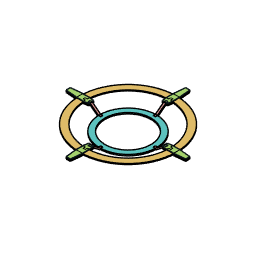
シロコ_ヘイロー_mk2 v9 (Autodesk Fusion 360 design; units mm, degrees)
Autodesk Fusion 360 part; units mm, degrees
sketch "スケッチ1" plane through (0, 0, 0) normal (0, 0, 1) x (1, 0, 0) in component "outer_ring"
  circle A0 centre (0, 0) radius 100
  circle A1 centre (0, 0) radius 116
  line L0 (-105, 2.5) -> (-105, -2.5)
  line L1 (0, 0) -> (-116, 0) construction
  line L2 (-105, 2.5) -> (-99.9687, 2.5)
  line L3 (-105, -2.5) -> (-99.9687, -2.5)
  line L4 (-2.5, -105) -> (-2.5, -99.9687)
  line L5 (-2.5, -105) -> (2.5, -105)
  line L6 (2.5, -105) -> (2.5, -99.9687)
  line L7 (105, -2.5) -> (99.9687, -2.5)
  line L8 (105, -2.5) -> (105, 2.5)
  line L9 (105, 2.5) -> (99.9687, 2.5)
  line L10 (2.5, 105) -> (2.5, 99.9687)
  line L11 (2.5, 105) -> (-2.5, 105)
  line L12 (-2.5, 105) -> (-2.5, 99.9687)
  point P0 (-100, 0)
  dimension "d1" = 200
  dimension "d2" = 232
  dimension "d14" = 5
  dimension "d15" = 5
  dimension "d17" = 360
  constraint coincident A0.centre A1.centre
  constraint concentric A0 A1
  constraint vertical L0
  constraint coincident A1 L1.end
  constraint perpendicular L0 L1
  constraint coincident A0 L2.end
  constraint perpendicular L0 L2
  constraint coincident A0 L3.end
  constraint perpendicular L0 L3
  constraint symmetric L1 L2 L3
  constraint coincident L1 P0
  constraint coincident A0 P0
  measures "d1" diameter of A0
  measures "d2" diameter of A1
  measures "d14" distance of L0.start L0.end
  measures "d15" distance of L0 P0
extrude "押し出し2" add sketch "スケッチ1" along normal blind 2 makes body 1 in component "outer_ring"
ref_plane "作業平面1" through (0, 0, -15) normal (0, 0, 1) x (1, 0, 0) in component "inner_ring"
sketch "スケッチ1 (2)" plane through (0, 0, -15) normal (0, 0, 1) x (1, 0, 0) in component "inner_ring"
  circle A0 centre (0, 0) radius 55
  circle A1 centre (0, 0) radius 68
  line L0 (0, 0) -> (-68, 0) construction
  line L1 (-63, 2.5) -> (-63, -2.5)
  line L2 (-63, 2.5) -> (-67.954, 2.5)
  line L3 (-63, -2.5) -> (-67.954, -2.5)
  line L4 (-2.5, -63) -> (-2.5, -67.954)
  line L5 (-2.5, -63) -> (2.5, -63)
  line L6 (2.5, -63) -> (2.5, -67.954)
  line L7 (63, -2.5) -> (67.954, -2.5)
  line L8 (63, -2.5) -> (63, 2.5)
  line L9 (63, 2.5) -> (67.954, 2.5)
  line L10 (2.5, 63) -> (2.5, 67.954)
  line L11 (2.5, 63) -> (-2.5, 63)
  line L12 (-2.5, 63) -> (-2.5, 67.954)
  dimension "d6" = 110
  dimension "d7" = 136
  dimension "d8" = 5
  dimension "d9" = 5
  dimension "d11" = 360
  constraint coincident A0.centre A1.centre
  constraint concentric A0 A1
  constraint coincident A1 L0.end
  constraint horizontal L0
  constraint perpendicular L0 L1
  constraint coincident A1 L2.end
  constraint perpendicular L1 L2
  constraint coincident A1 L3.end
  constraint perpendicular L1 L3
  constraint symmetric L0 L2 L3
  measures "d6" diameter of A0
  measures "d7" diameter of A1
  measures "d8" distance of L1.start L1.end
  measures "d9" distance of L0.end L1
extrude "押し出し1" add sketch "スケッチ1 (2)" along normal blind 2 separate body contours A1 L1 L2 L3 L4 L5 L6 L7 L8 L9 L10 L11 L12 makes body 2 in component "inner_ring"
sketch "スケッチ1 (3)" plane through (0, 0, 2) normal (0, 0, 1) x (-1, 0, 0) in component "protrusion_front"
  line L0 (2.5, -105) -> (-2.5, -105)
  line L1 (-2.5, -105) -> (-2.5, -99.9687)
  arc A0 (-99.9687, -2.5) -> (-2.5, -99.9687) centre (0, 0) ccw
  line L2 (-99.9687, -2.5) -> (-105, -2.5)
  line L3 (-105, -2.5) -> (-105, 2.5)
  line L4 (-105, 2.5) -> (-99.9687, 2.5)
  arc A1 (-2.5, 99.9687) -> (-99.9687, 2.5) centre (0, 0) ccw
  line L5 (-2.5, 99.9687) -> (-2.5, 105)
  line L6 (-2.5, 105) -> (2.5, 105)
  line L7 (2.5, 105) -> (2.5, 99.9687)
  arc A2 (99.9687, 2.5) -> (2.5, 99.9687) centre (0, 0) ccw
  line L8 (99.9687, 2.5) -> (105, 2.5)
  line L9 (105, 2.5) -> (105, -2.5)
  line L10 (105, -2.5) -> (99.9687, -2.5)
  arc A3 (2.5, -99.9687) -> (99.9687, -2.5) centre (0, 0) ccw
  line L11 (2.5, -99.9687) -> (2.5, -105)
  circle A4 centre (0, 0) radius 116
  line L12 (143, 0) -> (88, 0) construction
  line L13 (0, 0) -> (88, 0) construction
  circle A5 centre (0, 0) radius 116 construction
  circle A6 centre (0, 0) radius 100 construction
  line L14 (143, -5) -> (143, 5)
  line L15 (115.7573, -7.5) -> (115.7573, 7.5) construction
  line L16 (143, -5) -> (115.7573, -7.5)
  line L17 (143, 5) -> (115.7573, 7.5)
  line L18 (88, -6) -> (88, 6)
  line L19 (115.7573, -7.5) -> (99.7184, -7.5)
  line L20 (115.7573, 7.5) -> (99.7184, 7.5)
  line L21 (99.7184, 7.5) -> (88, 6)
  line L22 (99.7184, -7.5) -> (88, -6)
  line L23 (93, -2.5) -> (93, 2.5)
  line L24 (93, -2.5) -> (88, -2.5)
  line L25 (93, 2.5) -> (88, 2.5)
  circle A7 centre (0, 0) radius 99.75
  circle A8 centre (0, 0) radius 116.25
  line L26 (104.9, 2.4462) -> (104.9, -2.4538)
  line L27 (104.9, 2.4462) -> (99.72, 2.4462)
  line L28 (104.9, -2.4538) -> (99.7198, -2.4538)
  dimension "d20" = 55
  dimension "d21" = 88
  dimension "d22" = 232
  dimension "d23" = 200
  dimension "d24" = 10
  dimension "d25" = 15
  dimension "d26" = 12
  dimension "d27" = 5
  dimension "d28" = 5
  dimension "d29" = 199.5
  dimension "d30" = 232.5
  dimension "d33" = 4.9
  dimension "d37" = 104.9
  dimension "d38" = 5.18
  constraint horizontal L12
  constraint coincident A0.centre A1.centre
  constraint horizontal L13
  constraint coincident L12.end L13.end
  constraint concentric A0 A5
  constraint perpendicular L12 L14
  constraint midpoint L12.start L14
  constraint vertical L15
  constraint coincident A5 L15.start
  constraint symmetric L12 L15.start L15.end
  constraint vertical L18
  constraint midpoint L12.end L18
  constraint horizontal L19
  constraint coincident L15.start L16.end
  constraint coincident A6 L19.end
  constraint perpendicular L15 L20
  constraint coincident L15.end L17.end
  constraint coincident A6 L20.end
  constraint vertical L23
  constraint coincident L18 L24.end
  constraint perpendicular L18 L24
  constraint coincident L18 L25.end
  constraint perpendicular L18 L25
  constraint symmetric L12 L24 L25
  constraint concentric A6 A8
  constraint perpendicular L12 L26
  constraint coincident A7 L27.end
  constraint perpendicular L26 L27
  constraint perpendicular L26 L28
  constraint coincident A7 L28.end
  measures "d20" distance of L12.start L12.end
  measures "d21" distance of A0.centre L12.end
  measures "d22" diameter of A5
  measures "d23" diameter of A6
  measures "d24" distance of L14.start L14.end
  measures "d25" distance of L15.start L15.end
  measures "d26" distance of L18.start L18.end
  measures "d27" distance of L23.start L23.end
  measures "d28" distance of L23.start L24.end
  measures "d29" diameter of A7
  measures "d30" diameter of A8
  measures "d33" distance of L26.start L26.end
  measures "d37" distance of A0.centre L26
  measures "d38" distance of L26.start L27.end
extrude "押し出し2'" add sketch "スケッチ1 (3)" along normal blind 1 separate body contours A2 L8 L9 L10 A3 L21 L22 A7 L26 L27 L28 | A2 L8 L9 L10 A3 A4 L19 L20 | A4 L16 L17 A8 | L18 L21 L22 L23 L24 L25 A7 | L14 L16 L17 A8 | A7 L26 L27 L28 picked at (115.8862, 6.6596) makes body 3 in component "protrusion_front"
extrude "押し出し3" add sketch "スケッチ1 (3)" against normal blind 1 contours L18 L21 L22 L23 L24 L25 A7 | L14 L16 L17 A8 bodies 3 in component "protrusion_front"
extrude "押し出し4" add sketch "スケッチ1 (3)" against normal blind 2 contours A7 L26 L27 L28 bodies 3 in component "protrusion_front"
extrude "押し出し1'" add 2 faces at (-134.0744, -0.8313, 1) (-93.49, -5.3227, 1) along direction (0, 0, -1) blind 2 separate body on bodies 3 makes body 4 at (-134.0744, -0.8313, 1) makes body 5 at (-93.49, -5.3227, 1) in component "protrusion_back"
extrude "押し出し2''" cut 2 faces at (-134.0744, -0.8313, 1) (-93.49, -5.3227, 1) along direction (0, 0, -1) blind 1 on bodies 4 5 bodies 4 5 in component "protrusion_back"
loft "ロフト1" add section 1 face at (-99.7465, -0.8306, -0.6667) section 2 face at (-116.1044, -5.8169, -0.3333) on bodies 4 5 bodies 4 5 in component "protrusion_back"
extrude "押し出し3'" add 2 faces at (-134.0744, -0.8313, 1) (-93.49, -5.3227, 1) along direction (0, 0, -1) blind 1 on bodies 3 bodies 4 in component "protrusion_back"
move_body "移動1" bodies 3 to x (1, 0, 0) y (0, 1, 0) z (0, 0, 1) at (0, 0, 0.5) in component "protrusion_front"
extrude "押し出し5" add 2 faces at (-93.49, -5.3227, 1.5) (-134.0744, -0.8313, 1.5) along direction (0, 0, -1) blind 0.5 on bodies 3 bodies 3 in component "protrusion_front"
extrude "押し出し4'" add 2 faces at (-93.49, -5.3227, 1) (-134.0744, -0.8313, 1) along direction (0, 0, 1) blind 0.5 on bodies 4 bodies 4 in component "protrusion_back"
sketch "スケッチ1 (4)" plane through (0, 0, 3.5) normal (0, 0, 1) x (-1, 0, 0) in component "support"
  line L0 (93, -2.5) -> (88, -2.5)
  line L1 (88, -2.5) -> (88, -6)
  line L2 (88, -6) -> (99.7184, -7.5)
  line L3 (99.7184, -7.5) -> (115.7573, -7.5)
  line L4 (115.7573, -7.5) -> (143, -5)
  line L5 (143, -5) -> (143, 5)
  line L6 (143, 5) -> (115.7573, 7.5)
  line L7 (115.7573, 7.5) -> (99.7184, 7.5)
  line L8 (99.7184, 7.5) -> (88, 6)
  line L9 (88, 6) -> (88, 2.5)
  line L10 (88, 2.5) -> (93, 2.5)
  line L11 (93, 2.5) -> (93, -2.5)
  line L12 (93, -2.5) -> (88, -2.5)
  line L13 (88, -2.5) -> (88, 2.5)
  line L14 (88, 2.5) -> (93, 2.5)
  line L15 (93, 2.5) -> (93, -2.5)
  constraint horizontal L12
  constraint vertical L13
  constraint horizontal L14
  constraint vertical L15
  constraint coincident L9.end L10.start
  constraint coincident L0.start L11.end
sketch "スケッチ2" plane through (0, 0, -15) normal (0, 0, -1) x (1, 0, 0) in component "support"
  circle A0 centre (0, 0) radius 55
  line L0 (-2.5, -63) -> (2.5, -63)
  line L1 (2.5, -63) -> (2.5, -67.954)
  arc A1 (2.5, -67.954) -> (67.954, -2.5) centre (0, 0) ccw
  line L2 (67.954, -2.5) -> (63, -2.5)
  line L3 (63, -2.5) -> (63, 2.5)
  line L4 (63, 2.5) -> (67.954, 2.5)
  arc A2 (67.954, 2.5) -> (2.5, 67.954) centre (0, 0) ccw
  line L5 (2.5, 67.954) -> (2.5, 63)
  line L6 (2.5, 63) -> (-2.5, 63)
  line L7 (-2.5, 63) -> (-2.5, 67.954)
  arc A3 (-2.5, 67.954) -> (-67.954, 2.5) centre (0, 0) ccw
  line L8 (-67.954, 2.5) -> (-63, 2.5)
  line L9 (-63, 2.5) -> (-63, -2.5)
  line L10 (-63, -2.5) -> (-67.954, -2.5)
  arc A4 (-67.954, -2.5) -> (-2.5, -67.954) centre (0, 0) ccw
  line L11 (-2.5, -67.954) -> (-2.5, -63)
  line L12 (-67.954, 2.5) -> (-62.954, 2.5)
  line L13 (-62.954, 2.5) -> (-62.954, -2.5)
  line L14 (-62.954, -2.5) -> (-67.954, -2.5)
  line L15 (-67.954, -2.5) -> (-67.954, 2.5)
  dimension "d67" = 5
  dimension "d68" = 5
  constraint horizontal L12
  constraint vertical L13
  constraint horizontal L14
  constraint vertical L15
  constraint coincident A3.end L8.start
  measures "d67" distance of A3.end L12.end
  measures "d68" distance of A3.end L10.end
loft "ロフト1'" add profiles "スケッチ2", "スケッチ1 (4)" section 1 contours L8 L9 L10 L12 L14 L15 section 2 contours L0 L10 L11 L12 L13 L14 L15 separate body makes body 6 in component "support"
sketch "スケッチ1 (5)" plane through (0, 0, 3.5) normal (0, 0, 1) x (-1, 0, 0) in component "protrusion"
  line L0 (93, -2.5) -> (88, -2.5)
  line L1 (88, -2.5) -> (88, -6)
  line L2 (88, -6) -> (99.7184, -7.5)
  line L3 (99.7184, -7.5) -> (115.7573, -7.5)
  line L4 (115.7573, -7.5) -> (143, -5)
  line L5 (143, -5) -> (143, 5)
  line L6 (143, 5) -> (115.7573, 7.5)
  line L7 (115.7573, 7.5) -> (99.7184, 7.5)
  line L8 (99.7184, 7.5) -> (88, 6)
  line L9 (88, 6) -> (88, 2.5)
  line L10 (88, 2.5) -> (93, 2.5)
  line L11 (93, 2.5) -> (93, -2.5)
extrude "押し出し6" add sketch "スケッチ1 (3)" along normal up to surface (1.5 mm away) contours L18 L23 L24 L25 bodies 3 in component "protrusion_front"
extrude "押し出し7" cut 1 faces at (-89.6667, 0.8333, 2) along direction (0, 0, 1) blind 1 on bodies 3 bodies 3 in component "protrusion_front"
extrude "押し出し8" cut 1 faces at (-91.3333, 2.5, 1.6667) along direction (0, 1, 0) blind 0.05 on bodies 3 bodies 3 in component "protrusion_front"
extrude "押し出し9" cut 1 faces at (-89.6667, -2.5, 2.3333) along direction (0, -1, 0) blind 0.05 on bodies 3 bodies 3 in component "protrusion_front"
extrude "押し出し5'" cut 1 faces at (-89.6667, -2.5, -0.1667) along direction (0, -1, 0) blind 0.05 on bodies 4 bodies 4 in component "protrusion_back"
extrude "押し出し6'" cut 1 faces at (-89.6667, 2.5, -0.1667) along direction (0, 1, 0) blind 0.05 on bodies 4 bodies 4 in component "protrusion_back"
sketch "スケッチ1 (6)" plane through (0, 0, 0) normal (0, 1, 0) x (1, 0, 0) in component "pirrer"
  line L0 (-63, 13) -> (-63, 16)
  line L1 (-69.087, 16) -> (-63, 16)
  line L2 (-88, -2.3333) -> (-88, -3)
  line L3 (-88, -3) -> (-93, -3)
  line L4 (-93, -3) -> (-93, 1.5)
  line L5 (-63, 13) -> (-68, 13)
  line L6 (-93, 1.5) -> (-88, 1.5)
  line L7 (-88, 1.5) -> (-69.087, 16)
  line L8 (-88, -2.3333) -> (-68, 13)
  dimension "d88" = 3
  constraint perpendicular L3 L4
  constraint perpendicular L0 L5
  constraint parallel L7 L8
  measures "d88" distance of L0.start L0.end
extrude "押し出し1''" add sketch "スケッチ1 (6)" along normal blind 2.5 separate body makes body 7 in component "pirrer"
extrude "押し出し2'''" add 1 faces at (-81.3333, 0, -4.0556) along direction (0, -1, 0) blind 2.5 on bodies 7 bodies 7 in component "pirrer"
extrude "押し出し2''''" add 1 faces at (9.1157, -61.1473, -15) along direction (0, 0, -1) blind 1 on bodies 2 bodies 2 in component "inner_ring"
component_pattern "component pattern"
component "outer_ring" placed x (1, 0, 0) y (0, 1, 0) z (0, 0, 1) at (0, 0, 0)
component "inner_ring" placed x (1, 0, 0) y (0, 1, 0) z (0, 0, 1) at (0, 0, 0)
component "protrusion" placed x (1, 0, 0) y (0, 1, 0) z (0, 0, 1) at (0, 0, 0)
component "pirrer" placed x (1, 0, 0) y (0, 1, 0) z (0, 0, 1) at (0, 0, 0)
component "protrusion" placed x (0, 1, 0) y (-1, 0, 0) z (0, 0, 1) at (0, 0, 0)
component "pirrer" placed x (0, 1, 0) y (-1, 0, 0) z (0, 0, 1) at (0, 0, 0)
component "protrusion" placed x (-1, 0, 0) y (0, -1, 0) z (0, 0, 1) at (0, 0, 0)
component "pirrer" placed x (-1, 0, 0) y (0, -1, 0) z (0, 0, 1) at (0, 0, 0)
component "protrusion" placed x (0, -1, 0) y (1, 0, 0) z (0, 0, 1) at (0, 0, 0)
component "pirrer" placed x (0, -1, 0) y (1, 0, 0) z (0, 0, 1) at (0, 0, 0)
component "protrusion_front" placed x (1, 0, 0) y (0, 1, 0) z (0, 0, 1) at (0, 0, 0) in component "protrusion"
component "protrusion_back" placed x (1, 0, 0) y (0, 1, 0) z (0, 0, 1) at (0, 0, -0.5) in component "protrusion"
